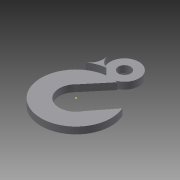
# Autodesk Inventor part: 4-5
Saved by Autodesk Inventor 2015 SP2 (Build 190223200, 223)
## iProperties
Created: 2015-09-21
Part Number: 4-5
Material: Generic
Document SubType Name: Modeling
Designer: KC-019
Density: 1 g/cm^3
Appearance: Default
Author: KC-019
Autodesk Inventor part; units mm, degrees
ref_plane "YZ Plane" through (0, 0, 0) normal (1, 0, 0) x (0, 1, 0)
ref_plane "XZ Plane" through (0, 0, 0) normal (0, 1, 0) x (-1, 0, 0)
ref_plane "XY Plane" through (0, 0, 0) normal (0, 0, 1) x (1, 0, 0)
sketch "Sketch1" plane through (0, 0, 0) normal (0, 0, 1) x (1, 0, 0)
  circle A0 centre (0, 0) radius 130
  circle A1 centre (0, 0) radius 62.5
  circle A2 centre (0, 180) radius 22.5
  circle A3 centre (0, 180) radius 53.5668
  arc A4 (-71.6362, 108.4816) -> (-51.3023, 164.5896) centre (-99.1885, 150.2053) ccw
  dimension "d0" = 260
  dimension "d1" = 125
  dimension "d2" = 45
  dimension "d4" = 180
  dimension "d5" = 100
  constraints: 3 centre point, 3 coincident, 2 point on circle, 8 other
  measures "d1" diameter of A1
  measures "d2" diameter of A2
  measures "d4" distance of point (0, 0) A2.centre
  measures "d5" diameter of A4
extrude "Extrusion1" add sketch "Sketch1" along normal blind 25 contours A0 A3 | A3 A0 | A0 A3
sketch "Sketch2" plane through (0, 0, 25) normal (0, 0, 1) x (1, 0, 0)
  arc A0 (-71.6362, 108.4816) -> (-51.3023, 164.5896) centre (-99.1885, 150.2053) ccw
  arc A1 (16.3015, 128.9739) -> (-16.3015, 128.9739) centre (0, 180) ccw projected
  arc A2 (-16.3015, 128.9739) -> (16.3015, 128.9739) centre (0, 0) ccw projected
  dimension "d8" = 100
  constraints: 4 point on circle, 2 tangent, 1 centre point
  measures "d8" diameter of A0
extrude "Extrusion2" add sketch "Sketch2" along normal blind 25 contours A0 A1 A2
sketch "Sketch3" plane through (0, 0, 25) normal (0, 0, 1) x (1, 0, 0)
  point P0 (0, 0)
sketch "Sketch4" plane through (0, 0, 25) normal (0, 0, 1) x (1, 0, 0)
  circle A0 centre (0, 0) radius 62.5 projected
  line L0 (-42.569, 45.7617) -> (89.7175, 203.6857)
  arc A1 (16.3015, 128.9739) -> (-51.3023, 164.5896) centre (0, 180) ccw projected
  line L1 (-42.569, 45.7617) -> (0, -2.5013)
  line L2 (0, -2.5013) -> (40.0872, -47.9506)
  line L3 (40.0872, -47.9506) -> (186.7208, 140.0495)
  line L4 (186.7208, 140.0495) -> (69.877, 180)
  constraints: 10 end point, 2 point on circle, 2 point on line, 1 tangent
extrude "Extrusion3" cut sketch "Sketch4" against normal blind 25 contours A0 L3 L2 L1 | A0 L0 L4 L3
sketch "Sketch5" plane through (0, 0, 25) normal (0, 0, 1) x (1, 0, 0)
  point P0 (0, 0)
body "Solid1"
